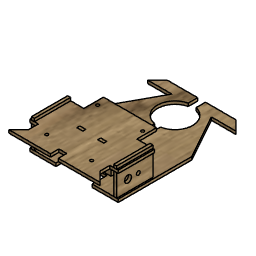
RC_Car_Formula-E (Autodesk Fusion 360 design; units mm, degrees)
Autodesk Fusion 360 part; units mm, degrees
sketch "Sketch1" plane through (0, 0, 0) normal (0, 0, 1) x (1, 0, 0)
  line L0 (90, 0) -> (90, 75.0046)
  line L1 (0, 75) -> (0, 0)
  line L2 (0, 0) -> (1.5, 0)
  line L3 (1.5, 0) -> (4.5, 0)
  line L4 (1.5, 12.25) -> (4.5, 12.25)
  line L5 (4.5, 12.25) -> (4.5, 6.25)
  line L6 (4.5, 6.25) -> (1.5, 6.25)
  line L7 (1.5, 6.25) -> (1.5, 12.25)
  line L8 (1.5, 12.25) -> (4.5, 6.25) construction
  line L9 (4.5, 12.25) -> (1.5, 6.25) construction
  line L10 (1.5, 30.75) -> (4.5, 30.75)
  line L11 (4.5, 30.75) -> (4.5, 24.75)
  line L12 (4.5, 24.75) -> (1.5, 24.75)
  line L13 (1.5, 24.75) -> (1.5, 30.75)
  line L14 (1.5, 30.75) -> (4.5, 24.75) construction
  line L15 (4.5, 30.75) -> (1.5, 24.75) construction
  line L16 (4.5, 6.25) -> (4.5, 12.25)
  line L17 (4.5, 24.75) -> (4.5, 30.75)
  line L18 (1.5, 30.75) -> (1.5, 24.75)
  line L19 (1.5, 12.25) -> (1.5, 6.25)
  line L20 (85.5, 12.25) -> (85.5, 6.25)
  line L21 (88.5, 6.25) -> (88.5, 12.25)
  line L22 (88.5, 12.25) -> (85.5, 12.25)
  line L23 (85.5, 6.25) -> (88.5, 6.25)
  line L24 (85.5, 24.75) -> (88.5, 24.75)
  line L25 (88.5, 30.75) -> (88.5, 24.75)
  line L26 (88.5, 30.75) -> (85.5, 30.75)
  line L27 (85.5, 24.75) -> (85.5, 30.75)
  line L28 (-50, 0) -> (-27.5, 0)
  line L29 (-27.5, 37) -> (-50, 37)
  line L30 (-27.5, 12.25) -> (-24.5, 12.25)
  line L31 (-24.5, 12.25) -> (-24.5, 6.25)
  line L32 (-24.5, 6.25) -> (-27.5, 6.25)
  line L33 (-27.5, 12.25) -> (-24.5, 6.25) construction
  line L34 (-24.5, 12.25) -> (-27.5, 6.25) construction
  line L35 (-27.5, 30.75) -> (-24.5, 30.75)
  line L36 (-24.5, 30.75) -> (-24.5, 24.75)
  line L37 (-24.5, 24.75) -> (-27.5, 24.75)
  line L38 (-27.5, 30.75) -> (-24.5, 24.75) construction
  line L39 (-24.5, 30.75) -> (-27.5, 24.75) construction
  line L40 (-27.5, 30.75) -> (-27.5, 37)
  line L41 (-27.5, 37) -> (-27.5, 30.75)
  line L42 (-24.5, 6.25) -> (-24.5, 12.25)
  line L43 (-24.5, 24.75) -> (-24.5, 30.75)
  line L44 (-27.5, 0) -> (-27.5, 6.25)
  line L45 (-27.5, 12.25) -> (-27.5, 24.75)
  line L46 (-27.5, 24.75) -> (-27.5, 12.25)
  line L47 (-27.5, 6.25) -> (-27.5, 0)
  line L48 (-53, 0) -> (-56, 0)
  line L49 (-56, 0) -> (-56, 37)
  line L50 (-56, 37) -> (-53, 37)
  line L51 (-50, 18.5) -> (-53, 18.5)
  circle A0 centre (-38.75, 11.5) radius 3.5
  circle A1 centre (-38.75, 22) radius 1.95
  line L52 (140, 0) -> (117.5, 0)
  line L53 (143, 0) -> (146, 0)
  line L54 (146, 37) -> (143, 37)
  line L55 (140, 18.5) -> (143, 18.5)
  line L56 (146, 0) -> (146, 37)
  line L57 (117.5, 30.75) -> (117.5, 37)
  line L58 (117.5, 37) -> (140, 37)
  line L59 (117.5, 24.75) -> (117.5, 12.25)
  line L60 (117.5, 12.25) -> (114.5, 12.25)
  line L61 (114.5, 6.25) -> (117.5, 6.25)
  line L62 (117.5, 0) -> (117.5, 6.25)
  line L63 (114.5, 6.25) -> (114.5, 12.25)
  line L64 (114.5, 24.75) -> (117.5, 24.75)
  line L65 (114.5, 30.75) -> (114.5, 24.75)
  line L66 (117.5, 30.75) -> (114.5, 30.75)
  circle A2 centre (128.75, 22) radius 1.95
  circle A3 centre (128.75, 11.5) radius 3.5
  line L67 (0, -27.2581) -> (81.5, -68.4462) construction
  line L68 (90, -27.2581) -> (8.5, -68.4462) construction
  line L69 (0, -26.5) -> (1.5, -26.5)
  line L70 (4.5, -26.5) -> (4.5, -45)
  line L71 (4.5, -45) -> (1.5, -45)
  line L72 (1.5, -45) -> (1.5, -26.5)
  line L73 (85.5, -26.5) -> (85.5, -45)
  line L74 (85.5, -45) -> (88.5, -45)
  line L75 (88.5, -45) -> (88.5, -26.5)
  line L76 (0, -26.5) -> (1.5, -26.5)
  line L77 (88.5, -26.5) -> (90, -26.5)
  line L78 (8.5, -73.5) -> (8.5, -63.5)
  line L79 (8.5, -63.5) -> (0, -63.5)
  line L80 (81.5, -73.5) -> (81.5, -63.5)
  line L81 (81.5, -63.5) -> (90, -63.5)
  line L82 (-1.5, -83.5) -> (8.5, -73.5)
  line L83 (91.5, -83.5) -> (81.5, -73.5)
  line L84 (89.989, 120.021) -> (64.9894, 120.021)
  line L85 (24.6387, 120.021) -> (0.011, 120.021)
  line L86 (0.011, 120.021) -> (9.994, 130.004)
  line L87 (0.011, 120.021) -> (14.1421, 120.021) construction
  line L88 (89.989, 120.021) -> (80.006, 130.004)
  line L89 (0, 75) -> (24.6387, 120.021)
  line L90 (90, 75.0046) -> (64.9894, 120.021)
  line L91 (26.5, 15) -> (63.5, 15)
  line L92 (63.5, 15) -> (63.5, 0)
  line L93 (26.5, 0) -> (26.5, 15)
  line L94 (0, 0) -> (26.5, 0)
  line L95 (63.5, 0) -> (90, 0)
  line L96 (-50, 0) -> (-50, 18.5)
  line L97 (-50, 18.5) -> (-53, 18.5)
  line L98 (-53, 18.5) -> (-53, 0)
  line L99 (-53, 37) -> (-50, 37)
  line L100 (140, 18.5) -> (143, 18.5)
  line L101 (143, 18.5) -> (143, 0)
  line L102 (140, 0) -> (140, 18.5)
  line L103 (140, 37) -> (143, 37)
  line L104 (72, -6.5) -> (18, -6.5)
  line L105 (18, -6.5) -> (18, -26.5)
  line L106 (72, -26.5) -> (72, -6.5)
  line L107 (72, -6.5) -> (18, -46.5) construction
  line L108 (18, -6.5) -> (72, -46.5) construction
  line L109 (4.5, -26.5) -> (18, -26.5)
  line L110 (72, -26.5) -> (85.5, -26.5)
  line L111 (31.375, 16.5) -> (37.375, 16.5)
  line L112 (37.375, 19.5) -> (31.375, 19.5)
  line L113 (31.375, 19.5) -> (31.375, 16.5)
  line L114 (31.375, 16.5) -> (37.375, 16.5)
  line L115 (37.375, 16.5) -> (37.375, 19.5)
  line L116 (37.375, 19.5) -> (31.375, 16.5) construction
  line L117 (31.375, 19.5) -> (37.375, 16.5) construction
  line L118 (58.625, 19.5) -> (52.625, 19.5)
  line L119 (52.625, 19.5) -> (52.625, 16.5)
  line L120 (52.625, 16.5) -> (58.625, 16.5)
  line L121 (58.625, 16.5) -> (58.625, 19.5)
  line L122 (58.625, 19.5) -> (52.625, 16.5) construction
  line L123 (52.625, 19.5) -> (58.625, 16.5) construction
  line L124 (58.625, 19.5) -> (52.625, 19.5)
  line L125 (37.375, 19.5) -> (31.375, 19.5)
  line L126 (23.75, -60.5) -> (23.75, -62)
  line L127 (37.375, -44) -> (31.375, -44)
  line L128 (31.375, -44) -> (31.375, -47)
  line L129 (31.375, -47) -> (37.375, -47)
  line L130 (37.375, -47) -> (37.375, -44)
  line L131 (37.375, -44) -> (31.375, -47) construction
  line L132 (31.375, -44) -> (37.375, -47) construction
  line L133 (58.625, -44) -> (52.625, -44)
  line L134 (52.625, -44) -> (52.625, -47)
  line L135 (52.625, -47) -> (58.625, -47)
  line L136 (58.625, -47) -> (58.625, -44)
  line L137 (58.625, -44) -> (52.625, -47) construction
  line L138 (52.625, -44) -> (58.625, -47) construction
  line L139 (58.625, -44) -> (52.625, -44)
  line L140 (31.375, -47) -> (37.375, -47)
  line L141 (52.625, -47) -> (58.625, -47)
  line L142 (24.2234, -60.5) -> (23.75, -60.5)
  line L143 (37.375, -44) -> (31.375, -44)
  line L144 (212.5, 0) -> (212.5, 22.5)
  line L145 (170, 22.5) -> (170, 0)
  line L146 (204.875, 25.5) -> (198.875, 25.5)
  line L147 (198.875, 25.5) -> (198.875, 22.5)
  line L148 (204.875, 22.5) -> (204.875, 25.5)
  line L149 (204.875, 25.5) -> (198.875, 22.5) construction
  line L150 (198.875, 25.5) -> (204.875, 22.5) construction
  line L151 (183.625, 25.5) -> (177.625, 25.5)
  line L152 (177.625, 25.5) -> (177.625, 22.5)
  line L153 (183.625, 22.5) -> (183.625, 25.5)
  line L154 (183.625, 25.5) -> (177.625, 22.5) construction
  line L155 (177.625, 25.5) -> (183.625, 22.5) construction
  line L156 (204.875, 25.5) -> (198.875, 25.5)
  line L157 (183.625, 25.5) -> (177.625, 25.5)
  line L158 (170, 22.5) -> (177.625, 22.5)
  line L159 (177.625, 22.5) -> (170, 22.5)
  line L160 (212.5, 22.5) -> (204.875, 22.5)
  line L161 (198.875, 22.5) -> (183.625, 22.5)
  line L162 (183.625, 22.5) -> (198.875, 22.5)
  line L163 (204.875, 22.5) -> (212.5, 22.5)
  line L164 (177.625, -3) -> (177.625, 0)
  line L165 (183.625, -3) -> (177.625, -3)
  line L166 (183.625, 0) -> (183.625, -3)
  line L167 (198.875, -3) -> (198.875, 0)
  line L168 (204.875, -3) -> (198.875, -3)
  line L169 (204.875, 0) -> (204.875, -3)
  line L170 (170, 0) -> (177.625, 0)
  line L171 (183.625, 0) -> (198.875, 0)
  line L172 (204.875, 0) -> (212.5, 0)
  circle A4 centre (67.9, -68.5) radius 1.5
  circle A5 centre (22.1, -68.5) radius 1.5
  circle A6 centre (67.9, -16.5) radius 1.5
  circle A7 centre (22.1, -16.5) radius 1.5
  line L173 (8.5, -63.5) -> (81.5, -63.5)
  line L174 (42, 85.1601) -> (42, 80.9084)
  line L175 (42, 80.9084) -> (48, 80.9084)
  line L176 (48, 80.9084) -> (48, 85.1601)
  line L177 (41, 130.004) -> (41, 120.4583)
  line L178 (49, 120.4583) -> (49, 130.004)
  line L179 (9.994, 130.004) -> (41, 130.004)
  line L180 (49, 130.004) -> (80.006, 130.004)
  arc A8 (41, 120.4583) -> (42, 85.1601) centre (45, 102.9084) ccw
  arc A9 (48, 85.1601) -> (49, 120.4583) centre (45, 102.9084) ccw
  line L181 (49, -75) -> (41, -75)
  line L182 (41, -75) -> (41, -83.5)
  line L183 (49, -83.5) -> (49, -75)
  line L184 (-1.5, -83.5) -> (41, -83.5)
  line L185 (49, -83.5) -> (91.5, -83.5)
  line L186 (90, -26.5) -> (90, -63.5)
  line L187 (0, -26.5) -> (0, -63.5)
  point P0 (3, 9.25)
  point P1 (3, 27.75)
  point P2 (45, -50)
  point P3 (45, -60.5)
  dimension "d1" = 90
  dimension "d3" = 1.5
  dimension "d4" = 3
  dimension "d6" = 3
  dimension "d7" = 6
  dimension "d8" = 6
  dimension "d11" = 36
  dimension "d12" = 22.5
  dimension "d13" = 37
  dimension "d15" = 6
  dimension "d16" = 6
  dimension "d17" = 6
  dimension "d19" = 7
  dimension "d21" = 3.9
  dimension "d26" = 3
  dimension "d27" = 18.5
  dimension "d35" = 45
  dimension "d36" = 90
  dimension "d41" = 54
  dimension "d42" = 40
  dimension "d47" = 6
  dimension "d48" = 3
  dimension "d49" = 6
  dimension "d53" = 6
  dimension "d54" = 3
  dimension "d55" = 6
  dimension "d56" = 3
  dimension "d57" = 42.5
  dimension "d58" = 22.5
  dimension "d59" = 42.5
  dimension "d61" = 6
  dimension "d62" = 6
  dimension "d65" = 3
  dimension "d66" = 3
  dimension "d67" = 52
  dimension "d68" = 3
  dimension "d69" = 3
  dimension "d72" = 16.5
  constraint horizontal L94
  constraint vertical L0
  constraint vertical L1
  constraint coincident L1.end L2.start
  constraint perpendicular L1 L2
  constraint horizontal L3
  constraint vertical L16
  constraint vertical L18
  constraint horizontal L4
  constraint perpendicular L4 L5
  constraint parallel L4 L6
  constraint parallel L5 L7
  constraint coincident L8 P0
  constraint coincident L9 P0
  constraint horizontal L10
  constraint perpendicular L10 L11
  constraint parallel L10 L12
  constraint parallel L11 L13
  constraint coincident L14 P1
  constraint coincident L15 P1
  constraint collinear L16 L17
  constraint collinear L18 L19
  constraint horizontal L28
  constraint vertical L44
  constraint horizontal L29
  constraint vertical L42
  constraint vertical L41
  constraint horizontal L30
  constraint perpendicular L30 L31
  constraint parallel L30 L32
  constraint horizontal L35
  constraint perpendicular L35 L36
  constraint parallel L35 L37
  constraint collinear L40 L44
  constraint collinear L41 L46
  constraint collinear L42 L43
  constraint collinear L44 L45
  constraint collinear L46 L47
  constraint horizontal L48
  constraint vertical L49
  constraint horizontal L50
  constraint horizontal L51
  constraint horizontal L76
  constraint coincident L67 P2
  constraint coincident L68 P2
  constraint vertical L70
  constraint horizontal L71
  constraint vertical L72
  constraint collinear L76 L109
  constraint collinear L77 L109
  constraint vertical L78
  constraint horizontal L79
  constraint vertical L80
  constraint horizontal L81
  constraint horizontal L184
  constraint perpendicular L82 L83
  constraint horizontal L179
  constraint horizontal L84
  constraint coincident L85.start L84
  constraint collinear L84 L85
  constraint horizontal L87
  constraint horizontal L91
  constraint perpendicular L91 L92
  constraint parallel L92 L93
  constraint coincident L92.end L94
  constraint collinear L94 L95
  constraint vertical L96
  constraint horizontal L97
  constraint vertical L98
  constraint horizontal L100
  constraint vertical L101
  constraint vertical L102
  constraint horizontal L104
  constraint perpendicular L104 L105
  constraint parallel L105 L106
  constraint coincident L106.start L109
  constraint collinear L109 L110
  constraint horizontal L124
  constraint parallel L111 L124
  constraint horizontal L112
  constraint perpendicular L112 L113
  constraint parallel L112 L114
  constraint parallel L113 L115
  constraint horizontal L118
  constraint perpendicular L118 L119
  constraint parallel L118 L120
  constraint parallel L119 L121
  constraint collinear L124 L125
  constraint horizontal L139
  constraint perpendicular L126 L139
  constraint parallel L139 L140
  constraint horizontal L127
  constraint perpendicular L127 L128
  constraint parallel L127 L129
  constraint parallel L128 L130
  constraint horizontal L133
  constraint perpendicular L133 L134
  constraint parallel L133 L135
  constraint parallel L134 L136
  constraint collinear L139 L143
  constraint collinear L140 L141
  constraint coincident L68 L142.start
  constraint horizontal L170
  constraint vertical L144
  constraint horizontal L160
  constraint vertical L145
  constraint horizontal L158
  constraint horizontal L156
  constraint horizontal L146
  constraint perpendicular L146 L147
  constraint parallel L147 L148
  constraint horizontal L151
  constraint perpendicular L151 L152
  constraint parallel L152 L153
  constraint collinear L156 L157
  constraint collinear L158 L162
  constraint collinear L159 L160
  constraint collinear L160 L161
  constraint collinear L162 L163
  constraint collinear L170 L171
  constraint collinear L171 L172
  constraint coincident L78 L68.end
  constraint coincident L80 L67.end
  constraint perpendicular L80 L173
  constraint parallel L174 L176
  constraint parallel L177 L178
  constraint collinear L179 L180
  constraint concentric A8 A9
  constraint horizontal L181
  constraint perpendicular L181 L182
  constraint parallel L182 L183
  constraint collinear L184 L185
  constraint perpendicular L81 L186
  constraint perpendicular L79 L187
  constraint coincident L186 L68.start
  constraint coincident L187 L67.start
  measures "d1" distance of L1.end L0.start
  measures "d3" distance of L1.end L2.end
  measures "d4" distance of L2.end L3.end
  measures "d6" distance of L5.end L6.end
  measures "d7" distance of L4.end L5.end
  measures "d8" distance of L10.end L11.end
  measures "d11" diameter of A8
  measures "d12" distance of L28.start L28.end
  measures "d13" distance of L28.start L29.end
  measures "d15" distance of L30.end L31.end
  measures "d16" distance of L35.end L36.end
  measures "d17" distance of L28.start L48.end
  measures "d19" diameter of A0
  measures "d21" diameter of A1
  measures "d26" distance of L69.end L70.start
  measures "d27" distance of L69.end L71.end
  measures "d35" angle of L86 L87
  measures "d36" angle of L86 L88
  measures "d41" distance of L107.end L108.end
  measures "d42" distance of L104.end L107.end
  measures "d47" distance of L111.start L111.end
  measures "d48" distance of L112.end L111.start
  measures "d49" distance of L119.end L120.end
  measures "d53" distance of L128.end L129.end
  measures "d54" distance of L127.end L128.end
  measures "d55" distance of L134.end L135.end
  measures "d56" distance of L133.end L134.end
  measures "d57" distance of L145.end L144.start
  measures "d58" distance of L145.end L145.start
  measures "d59" distance of L145.start L144.end
  measures "d61" distance of L147.end L148.start
  measures "d62" distance of L152.end L153.start
  measures "d65" diameter of A4
  measures "d66" diameter of A5
  measures "d67" distance of A5.centre A7.centre
  measures "d68" diameter of A6
  measures "d69" diameter of A7
  measures "d72" distance of L140 L173
extrude "Extrude1" [suppressed]
extrude "Extrude2" add sketch "Sketch1" along normal blind 3 makes body 1 at (-38.7014, 32.6482, 0) makes body 2 at (47.5417, -25.9757, 0) makes body 3 at (128.7986, 32.6482, 0) makes body 4 at (74.5, 62.221, 0) makes body 5 at (193.7917, 7.5, 0)
move_body "Move1" bodies 3 to x (1, 0, 0) y (0, 1, 0) z (0, 0, 1) at (-26, 0, 0)
move_body "Move2" bodies 3 to x (0, 0, 1) y (0, 1, 0) z (-1, 0, 0) at (88.5, 0, -88.5)
move_body "Move3" bodies 1 to x (0, 0, -1) y (0, 1, 0) z (1, 0, 0) at (-40.25, 0, -40.25)
move_body "Move4" bodies 1 to x (1, 0, 0) y (0, 1, 0) z (0, 0, 1) at (41.75, 0, 15.75)
move_body "Move5" bodies 5 to x (1, 0, 0) y (0, 0, 1) z (0, -1, 0) at (0, 0, 0)
move_body "Move6" bodies 5 to x (1, 0, 0) y (0, 1, 0) z (0, 0, 1) at (-146.25, 19.5, 3)
move_body "Move7" bodies 2 to x (1, 0, 0) y (0, 1, 0) z (0, 0, 1) at (0, 63.5, 25.5)
